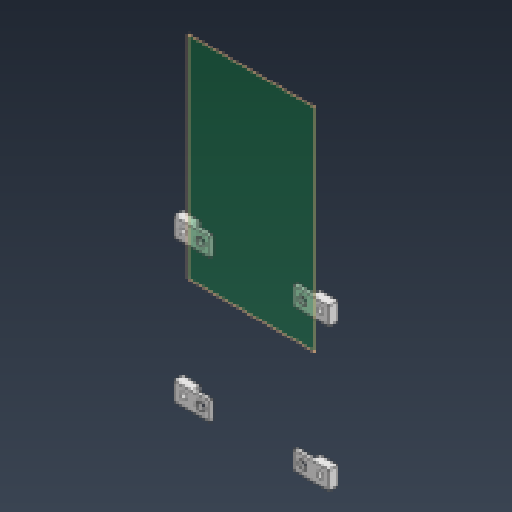
# Autodesk Inventor part: BMS_hold_check
Saved by Autodesk Inventor 2023 (Build 270158000, 158)
## iProperties
Created: 2025-12-27
Part Number: BMS_hold_check
Material: Generic
Document SubType Name: Modeling
Designer: szymo
Density: 1 g/cm^3
Appearance: Default
Author: szymo
Autodesk Inventor part; units mm, degrees
ref_plane "YZ Plane" through (0, 0, 0) normal (1, 0, 0) x (0, 1, 0)
ref_plane "XZ Plane" through (0, 0, 0) normal (0, 1, 0) x (-1, 0, 0)
ref_plane "XY Plane" through (0, 0, 0) normal (0, 0, 1) x (1, 0, 0)
ref_plane "Work Plane1" through (0, 5.7871, -6) normal (0, 0, -1) x (-1, 0, 0)
sketch "Sketch1" plane through (0, 5.7871, -6) normal (0, 0, -1) x (-1, 0, 0)
  circle A0 centre (-28.5, -38.0871) radius 2.075 projected
  circle A1 centre (-28.5, -117.9871) radius 2.075 projected
  circle A2 centre (28.5, -38.0871) radius 2.075 projected
  circle A3 centre (28.5, -117.9871) radius 2.075 projected
  line L0 (-30.2, -121.9121) -> (30.2, -121.9121) projected
  arc A4 (30.2, -121.9121) -> (32.5, -119.6121) centre (30.2, -119.6121) ccw projected
  line L1 (32.5, -119.6121) -> (32.5, -16.2121) projected
  arc A5 (32.5, -16.2121) -> (30.2, -13.9121) centre (30.2, -16.2121) ccw projected
  line L2 (30.2, -13.9121) -> (-30.2, -13.9121) projected
  arc A6 (-30.2, -13.9121) -> (-32.5, -16.2121) centre (-30.2, -16.2121) ccw projected
  line L3 (-32.5, -16.2121) -> (-32.5, -119.6121) projected
  arc A7 (-32.5, -119.6121) -> (-30.2, -121.9121) centre (-30.2, -119.6121) ccw projected
  line L4 (43.575, -123.0621) -> (23.425, -123.0621)
  line L5 (23.425, -123.0621) -> (23.425, -112.9121)
  line L6 (23.425, -112.9121) -> (43.575, -112.9121)
  line L7 (43.575, -112.9121) -> (43.575, -123.0621)
  line L8 (-43.575, -123.0621) -> (-23.425, -123.0621)
  line L9 (-23.425, -123.0621) -> (-23.425, -112.9121)
  line L10 (-23.425, -112.9121) -> (-43.575, -112.9121)
  line L11 (-43.575, -112.9121) -> (-43.575, -123.0621)
  line L12 (-43.575, -43.1621) -> (-23.425, -43.1621)
  line L13 (-23.425, -43.1621) -> (-23.425, -33.0121)
  line L14 (-23.425, -33.0121) -> (-43.575, -33.0121)
  line L15 (-43.575, -33.0121) -> (-43.575, -43.1621)
  line L16 (43.575, -43.1621) -> (23.425, -43.1621)
  line L17 (23.425, -43.1621) -> (23.425, -33.0121)
  line L18 (23.425, -33.0121) -> (43.575, -33.0121)
  line L19 (43.575, -33.0121) -> (43.575, -43.1621)
  circle A8 centre (28.5, -117.9871) radius 5.075
  circle A9 centre (-28.5, -117.9871) radius 5.075
  circle A10 centre (28.5, -38.0871) radius 5.075
  circle A11 centre (-28.5, -38.0871) radius 5.075
  line L20 (33.575, -33.0121) -> (33.575, -43.1621)
  line L21 (-33.575, -33.0121) -> (-33.575, -43.1621)
  line L22 (-33.575, -112.9121) -> (-33.575, -123.0621)
  line L23 (33.5, -112.9121) -> (33.5, -123.0621)
  point P0 (0, -5.7871)
  dimension "d0" = 3
  dimension "d1" = 3
  dimension "d2" = 3
  dimension "d3" = 3
  dimension "d5" = 10
  dimension "d6" = 10
  dimension "d7" = 10
  dimension "d8" = 10
  constraints: 40 end point, 14 tangent, 8 parallel, 7 perpendicular, 7 point on line, 4 centre point, 4 horizontal, 2 midpoint
  measures "d0" radial gap between concentric circles of A3 A8
  measures "d1" radial gap between concentric circles of A1 A9
  measures "d2" radial gap between concentric circles of A2 A10
  measures "d3" radial gap between concentric circles of A0 A11
  measures "d5" distance edge to line of A8 L7
  measures "d6" distance edge to line of A9 L11
  measures "d7" distance edge to line of A11 L15
  measures "d8" distance edge to line of A10 L19
extrude "Extrusion1" add sketch "Sketch1" along normal blind 2 contours A0 | A1 | A2 | A3 | A7 L3 A9 L0 | L0 A9 L3 A7 | A9 L9 L0 | L0 L9 L8 A9 | L8 L22 A9 | A9 L10 L9 | A9 L22 L10 L3 | L3 L10 A9 | L5 A8 L0 | L0 A8 L4 L5 | L8 L11 L10 L22 | A8 L1 A4 L0 | L0 A4 L1 A8 L23 | L5 L6 A8 | L12 L21 A11 L3 | L3 A11 L12 | A8 L23 L4 | L6 L1 A8 | A11 L3 | L3 A11 | L12 L15 L14 L21 | A11 L13 L12 | L23 A8 L6 L7 L4 | L23 A8 | L6 L23 A8 L1 | A11 L21 L14 L3 | L3 L14 A11 | A11 L14 L13 | L16 A10 L1 | L1 A10 L20 L16 | A10 L1 | L1 A10 | L20 L18 L19 L16 | L16 L17 A10 | A10 L18 L1 | L1 L18 L20 A10 | L17 L18 A10
sketch "Sketch3" plane through (0, 5.7871, -8) normal (0, 0, -1) x (-1, 0, 0)
  circle A0 centre (-28.5, -38.0871) radius 2.075 projected
  circle A1 centre (28.5, -38.0871) radius 2.075 projected
  circle A2 centre (28.5, -117.9871) radius 2.075 projected
  circle A3 centre (-28.5, -117.9871) radius 2.075 projected
  point P0 (0, -5.7871)
extrude "Extrusion3" cut sketch "Sketch3" against normal through all
chamfer "Chamfer1" distance 0.5 angle 45 4 edges at (30.575, -32.3, -6) (-26.425, -32.3, -6) (-26.425, -112.2, -6) (30.575, -112.2, -6)
sketch "Sketch6" plane through (0, 5.7871, -8) normal (0, 0, -1) x (-1, 0, 0)
  circle A0 centre (28.5, -38.0871) radius 2.075 projected
  line L0 (43.575, -33.0121) -> (23.425, -33.0121) projected
  line L1 (23.425, -33.0121) -> (23.425, -43.1621) projected
  line L2 (23.425, -43.1621) -> (43.575, -43.1621) projected
  line L3 (43.575, -43.1621) -> (43.575, -33.0121) projected
  circle A1 centre (-28.5, -38.0871) radius 2.075 projected
  line L4 (-23.425, -43.1621) -> (-23.425, -33.0121) projected
  line L5 (-23.425, -33.0121) -> (-43.575, -33.0121) projected
  line L6 (-43.575, -33.0121) -> (-43.575, -43.1621) projected
  line L7 (-43.575, -43.1621) -> (-23.425, -43.1621) projected
  circle A2 centre (28.5, -117.9871) radius 2.075 projected
  line L8 (43.575, -112.9121) -> (23.425, -112.9121) projected
  line L9 (23.425, -112.9121) -> (23.425, -123.0621) projected
  line L10 (23.425, -123.0621) -> (43.575, -123.0621) projected
  line L11 (43.575, -123.0621) -> (43.575, -112.9121) projected
  circle A3 centre (-28.5, -117.9871) radius 2.075 projected
  line L12 (-43.575, -123.0621) -> (-23.425, -123.0621) projected
  line L13 (-23.425, -123.0621) -> (-23.425, -112.9121) projected
  line L14 (-23.425, -112.9121) -> (-43.575, -112.9121) projected
  line L15 (-43.575, -112.9121) -> (-43.575, -123.0621) projected
  line L16 (43.575, -123.0621) -> (33.575, -123.0621)
  line L17 (33.575, -123.0621) -> (33.575, -112.9121)
  line L18 (33.575, -112.9121) -> (43.575, -112.9121)
  line L19 (43.575, -112.9121) -> (43.575, -123.0621)
  line L20 (-43.575, -123.0621) -> (-33.575, -123.0621)
  line L21 (-33.575, -123.0621) -> (-33.575, -112.9121)
  line L22 (-33.575, -112.9121) -> (-43.575, -112.9121)
  line L23 (-43.575, -112.9121) -> (-43.575, -123.0621)
  line L24 (43.575, -43.1621) -> (33.575, -43.1621)
  line L25 (33.575, -43.1621) -> (33.575, -33.0121)
  line L26 (33.575, -33.0121) -> (43.575, -33.0121)
  line L27 (43.575, -33.0121) -> (43.575, -43.1621)
  line L28 (-23.425, -43.1621) -> (-33.425, -43.1621)
  line L29 (-33.425, -43.1621) -> (-33.425, -33.0121)
  line L30 (-33.425, -33.0121) -> (-23.425, -33.0121)
  line L31 (-23.425, -33.0121) -> (-23.425, -43.1621)
  point P0 (0, -5.7871)
  point P1 (33.575, -112.9121)
  point P2 (33.575, -33.0121)
  point P3 (33.575, -43.1621)
  point P4 (-33.425, -33.0121)
  point P5 (-33.575, -112.9121)
  dimension "d46" = 10
  dimension "d47" = 10.15
  dimension "d48" = 10
  dimension "d49" = 10.15
  dimension "d50" = 10
  dimension "d51" = 10.15
  dimension "d52" = 10
  dimension "d53" = 10.15
  constraints: 32 end point, 8 parallel, 4 horizontal, 4 perpendicular
  measures "d46" distance of L17.end L18.end
  measures "d47" distance of L16.end L17.end
  measures "d48" distance of L22.end L21.end
  measures "d49" distance of L21.end L20.end
  measures "d50" distance of L25.end L26.end
  measures "d51" distance of L24.end L25.end
  measures "d52" distance of L29.end L30.end
  measures "d53" distance of L28.end L29.end
extrude "Extrusion5" add sketch "Sketch6" along normal blind 3 contours L3 L2 L25 L0 | L7 L6 L5 L29 | L11 L10 L17 L8 | L15 L14 L21 L12
sketch "Sketch7" plane through (0, 5.7871, -11) normal (0, 0, -1) x (-1, 0, 0)
  line L0 (33.575, -123.0621) -> (43.575, -123.0621) projected
  line L1 (43.575, -123.0621) -> (43.575, -112.9121) projected
  line L2 (43.575, -112.9121) -> (33.575, -112.9121) projected
  line L3 (-33.575, -112.9121) -> (-43.575, -112.9121) projected
  line L4 (-43.575, -112.9121) -> (-43.575, -123.0621) projected
  line L5 (-43.575, -123.0621) -> (-33.575, -123.0621) projected
  line L6 (-33.575, -123.0621) -> (-33.575, -112.9121) projected
  line L7 (-43.575, -43.1621) -> (-33.425, -43.1621) projected
  line L8 (-33.425, -43.1621) -> (-33.425, -33.0121) projected
  line L9 (-33.425, -33.0121) -> (-43.575, -33.0121) projected
  line L10 (-43.575, -33.0121) -> (-43.575, -43.1621) projected
  line L11 (33.575, -43.1621) -> (43.575, -43.1621) projected
  line L12 (43.575, -43.1621) -> (43.575, -33.0121) projected
  line L13 (43.575, -33.0121) -> (33.575, -33.0121) projected
  line L14 (23.425, -123.0621) -> (43.575, -123.0621) projected
  line L15 (43.575, -123.0621) -> (33.0445, -112.6955)
  line L16 (-43.575, -123.0621) -> (-23.425, -123.0621) projected
  line L17 (-43.575, -123.0621) -> (-33.5, -112.9121)
  line L18 (-23.425, -112.9121) -> (-43.575, -112.9121) projected
  line L19 (-43.575, -33.0121) -> (-43.575, -43.1621) projected
  line L20 (-43.575, -33.0121) -> (-33.425, -43.0871)
  line L21 (43.575, -43.1621) -> (43.575, -33.0121) projected
  line L22 (43.575, -33.0121) -> (33.5, -43.1621)
  line L23 (23.425, -43.1621) -> (43.575, -43.1621) projected
  line L24 (33.575, -33.0121) -> (43.8006, -43.1621)
  line L25 (43.575, -123.0621) -> (43.575, -112.9121) projected
  line L26 (-43.575, -112.9121) -> (-43.575, -123.0621) projected
  line L27 (-43.575, -112.9121) -> (-33.575, -123.0621)
  line L28 (-23.425, -33.0121) -> (-43.575, -33.0121) projected
  line L29 (-33.2728, -33.0121) -> (-43.575, -43.1621)
  line L30 (33.575, -33.0121) -> (33.575, -43.1621) projected
  line L31 (33.575, -112.9121) -> (33.575, -123.0621) projected
  point P0 (0, -5.7871)
  point P1 (33.575, -37.375)
  point P2 (38.3097, -117.8788)
  point P3 (-38.575, -117.9871)
  point P4 (-38.4239, -38.0871)
  point P5 (38.6878, -38.0871)
  constraints: 14 end point, 5 midpoint, 4 perpendicular, 3 point on line, 2 other
hole "Hole2" at (-38.3097, -112.0917, -11) at (38.575, -112.2, -11) at (38.4239, -32.3, -11) at (-38.6878, -32.3, -11) direction (0, 0, 1) diameter 3.6 depth 15 countersink diameter 7 countersink angle 90 clearance for "Countersunk Flat Head Screw ISO 2009/7046" size "M3" standard "ISO"
equation "\"d1\" = d0"
equation "\"d2\" = d0"
equation "\"d3\" = d0"
equation "\"d6\" = d5"
equation "\"d7\" = d5"
equation "\"d8\" = d5"
body "Solid1"
